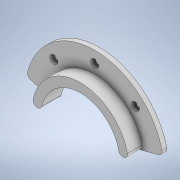
# Autodesk Inventor part: HoseClampShaftCollarShooterMount
Saved by Autodesk Inventor 2020 (Build 240168000, 168)
## iProperties
Created: 2020-01-29
Part Number: HoseClampShaftCollarShooterMount
Material: Generic
Document SubType Name: Modeling
Designer: srini
Density: 1 g/cm^3
Appearance: Default
Author: srini
Autodesk Inventor part; units mm, degrees
ref_plane "YZ Plane" through (0, 0, 0) normal (1, 0, 0) x (0, 1, 0)
ref_plane "XZ Plane" through (0, 0, 0) normal (0, 1, 0) x (-1, 0, 0)
ref_plane "XY Plane" through (0, 0, 0) normal (0, 0, 1) x (1, 0, 0)
sketch "Sketch1" plane through (0, 0, 0) normal (0, 0, 1) x (1, 0, 0)
  arc A0 (28.3106, 6.35) -> (-28.3106, 6.35) centre (0, 0) ccw construction
  arc A1 (31.1988, 6.9978) -> (-31.1988, 6.9978) centre (0, 0) ccw
  arc A2 (25.4224, 5.7022) -> (-25.4224, 5.7022) centre (0, 0) ccw
  arc A3 (25.4224, 5.7022) -> (31.1988, 6.9978) centre (28.3106, 6.35) ccw
  arc A4 (-31.1988, 6.9978) -> (-25.4224, 5.7022) centre (-28.3106, 6.35) ccw
  dimension "d0" = 2.96
  dimension "d1" = 26.054
  dimension "d2" = 6.35
  dimension "d5" = 31.974
  constraints: 10 point on circle, 5 centre point, 4 tangent, 1 coincident, 1 horizontal alignment
  measures "d0" radius of A4
  measures "d1" radius of A2
  measures "d2" vertical distance of point (0, 0) A0.end
  measures "d5" radius of A1
extrude "Extrusion1" add sketch "Sketch1" along normal blind 12.7
sketch "Sketch2" plane through (0, 0, 0) normal (0, 0, -1) x (-1, 0, 0)
  arc A0 (31.1988, 6.9978) -> (-31.1988, 6.9978) centre (0, 0) ccw projected
  arc A1 (44.3474, 11.1189) -> (-44.4956, 10.5098) centre (0, 0) ccw
  arc A2 (-44.4956, 10.5098) -> (-42.3638, 6.9657) centre (-41.6149, 9.8294) ccw
  line L0 (-42.3638, 6.9657) -> (-29.0595, 3.4863)
  arc A3 (-31.1988, 6.9978) -> (-25.4224, 5.7022) centre (-28.3106, 6.35) ccw projected
  arc A4 (25.4224, 5.7022) -> (31.1988, 6.9978) centre (28.3106, 6.35) ccw projected
  line L1 (29.1807, 3.5208) -> (42.3463, 7.5698)
  arc A5 (42.3463, 7.5698) -> (44.3474, 11.1189) centre (41.4762, 10.3991) ccw
  arc A6 (-31.1988, 6.9978) -> (-25.4224, 5.7022) centre (-28.3106, 6.35) ccw projected
  dimension "d6" = 45.72
  constraints: 8 point on circle, 6 tangent, 4 end point, 3 centre point, 2 equal radius
  measures "d6" radius of A1
extrude "Extrusion2" add sketch "Sketch2" against normal blind 3.175
sketch "Sketch3" plane through (0, 0, 3.175) normal (0, 0, 1) x (1, 0, 0)
  circle A0 centre (-26.9408, 26.9408) radius 2.667
  line L0 (0, 0) -> (0, 4.8755)
  circle A1 centre (0, 38.1) radius 2.667
  circle A2 centre (26.9408, 26.9408) radius 2.667
  dimension "d9" = 5.334
  dimension "d10" = 38.1
  dimension "d11" = 45
  dimension "d14" = 90
  constraints: 3 centre point, 2 end point, 1 vertical, 5 other
  measures "d9" diameter of A0
  measures "d10" distance of L0.start A0.centre
extrude "Extrusion3" cut sketch "Sketch3" against normal through all
body "Solid1"
